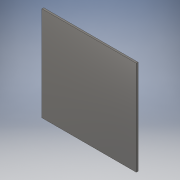
# Autodesk Inventor part: Rear
Saved by Autodesk Inventor 2017 (Build 210142000, 142)
## iProperties
Created: 2017-01-03
Part Number: Rear
Material: Steel, Mild
Document SubType Name: Sheet Metal
Designer: Robert.Chapman
Density: 7.85 g/cm^3
Sheet Metal Rule: Default
Appearance: Semi-Polished
Author: Robert.Chapman
Autodesk Inventor part; units mm, degrees
ref_plane "YZ Plane" through (0, 0, 0) normal (1, 0, 0) x (0, 1, 0)
ref_plane "XZ Plane" through (0, 0, 0) normal (0, 1, 0) x (-1, 0, 0)
ref_plane "XY Plane" through (0, 0, 0) normal (0, 0, 1) x (1, 0, 0)
sketch "Sketch1" plane through (0, 0, 0) normal (0, 0, 1) x (1, 0, 0)
  line L0 (-127, -127) -> (127, -127)
  line L1 (127, -127) -> (127, 127)
  line L2 (127, 127) -> (-127, 127)
  line L3 (-127, 127) -> (-127, -127)
  line L4 (-127, -127) -> (127, 127) construction
  line L5 (127, -127) -> (-127, 127) construction
  point P0 (0, 0)
  dimension "d0" = 254
  dimension "d1" = 254
  measures "d0" distance of L1.end L2.end
  measures "d1" distance of L0.end L1.end
extrude "Plate1" add sketch "Sketch1" along normal blind 4.7625
equation "\"BendRadius\" = Thickness"
equation "\"BendReliefWidth\" = Thickness"
equation "\"BendReliefDepth\" = 0.5 * Thickness"
equation "\"CornerReliefSize\" = 4 * Thickness"
equation "\"MinimumRemnant\" = 2 * Thickness"
equation "\"TransitionRadius\" = BendRadius"
equation "\"JacobiRadiusSize\" = BendRadius"
equation "\"GapSize\" = Thickness"
equation "\"d2\" = BendRadius"
equation "\"Thickness\" = 4.7625"
body "Solid1"
